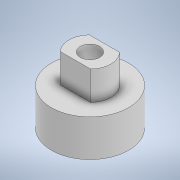
# Autodesk Inventor part: axle extender
Saved by Autodesk Inventor 2020.1 (Build 241239000, 239)
## iProperties
Created: 2019-10-24
Part Number: axle extender
Material: Generic
Document SubType Name: Modeling
Designer: amirs
Density: 1 g/cm^3
Appearance: Default
Author: amirs
Autodesk Inventor part; units mm, degrees
ref_plane "YZ Plane" through (0, 0, 0) normal (1, 0, 0) x (0, 1, 0)
ref_plane "XZ Plane" through (0, 0, 0) normal (0, 1, 0) x (-1, 0, 0)
ref_plane "XY Plane" through (0, 0, 0) normal (0, 0, 1) x (1, 0, 0)
sketch "Sketch1" plane through (0, 0, 0) normal (0, 1, 0) x (-1, 0, 0)
  circle A0 centre (0, 0) radius 6.096
  line L0 (3.81, 0) -> (-3.81, 0) construction
  line L1 (2.5903, -2.794) -> (-2.5903, -2.794)
  line L2 (2.5903, 2.794) -> (-2.5903, 2.794)
  arc A1 (-2.5903, 2.794) -> (-2.5903, -2.794) centre (0, 0) ccw
  arc A2 (2.5903, -2.794) -> (2.5903, 2.794) centre (0, 0) ccw
  dimension "d0" = 12.192
  dimension "d2" = 5.588
  dimension "d3" = 2.794
  dimension "d13" = 3.81
  dimension "d14" = 3.81
  constraints: 6 end point, 6 point on circle, 3 centre point, 3 horizontal, 2 coincident, 1 horizontal alignment
  measures "d0" diameter of A0
  measures "d2" distance between parallel lines of L2 L1
  measures "d3" distance between parallel lines of L0 L1
  measures "d13" radius of A1
  measures "d14" radius of A2
extrude "Extrusion1" add sketch "Sketch1" along normal blind 5.08
sketch "Sketch2" plane through (0, 5.08, 0) normal (0, 1, 0) x (1, 0, 0)
  circle A0 centre (0, 0) radius 6.096
  constraints: 1 centre point, 1 coincident
extrude "Extrusion2" add sketch "Sketch2" along normal blind 0.762
sketch "Sketch3" plane through (0, 5.842, 0) normal (0, 1, 0) x (1, 0, 0)
  arc A0 (-2.5903, 2.794) -> (-2.5903, -2.794) centre (0, 0) ccw construction
  arc A1 (-2.5903, 2.794) -> (-2.5903, -2.794) centre (0, 0) ccw projected
  line L0 (-2.5903, 2.794) -> (2.5903, 2.794) construction
  line L1 (-2.5903, 2.794) -> (2.5903, 2.794) projected
  arc A2 (2.5903, -2.794) -> (2.5903, 2.794) centre (0, 0) ccw construction
  arc A3 (2.5903, -2.794) -> (2.5903, 2.794) centre (0, 0) ccw projected
  line L2 (2.5903, -2.794) -> (-2.5903, -2.794) construction
  line L3 (2.5903, -2.794) -> (-2.5903, -2.794) projected
  arc A4 (-2.3827, 2.286) -> (-2.3827, -2.286) centre (0, 0) ccw
  line L4 (-2.3827, 2.286) -> (2.3827, 2.286)
  arc A5 (2.3827, -2.286) -> (2.3827, 2.286) centre (0, 0) ccw
  line L5 (2.3827, -2.286) -> (-2.3827, -2.286)
  point P0 (-2.5903, -2.794)
  dimension "d15" = 0.508
  dimension "d16" = 0.508
  dimension "d17" = 0.508
  dimension "d18" = 0.508
  constraints: 4 end point, 4 point on circle, 2 centre point, 2 parallel
  measures "d15" radial gap between concentric circles of A0 A4
  measures "d16" distance between parallel lines of L0 L4
  measures "d17" radial gap between concentric circles of A2 A5
  measures "d18" distance between parallel lines of L2 L5
extrude "Extrusion3" add sketch "Sketch3" along normal blind 4.572 contours L4 A5 L5 A4
sketch "Sketch4" plane through (0, 10.414, 0) normal (0, 1, 0) x (1, 0, 0)
  circle A0 centre (0, 0) radius 1.524
  dimension "d10" = 3.048
  constraints: 1 centre point, 1 coincident
  measures "d10" diameter of A0
extrude "Extrusion4" cut sketch "Sketch4" against normal blind 25.4
equation "\"d3\" = 0.5 * d2"
body "Solid1"
